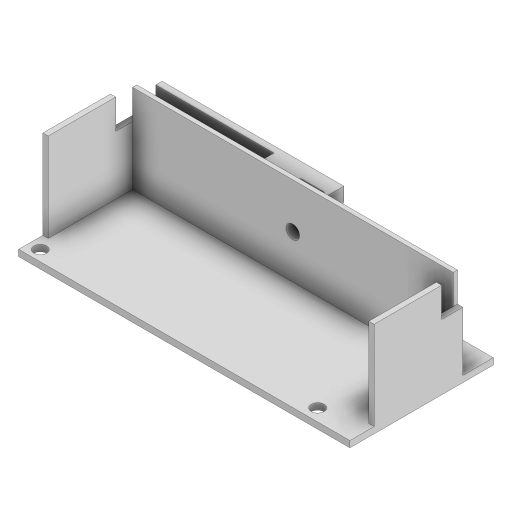
# Autodesk Inventor part: Part2
Saved by Autodesk Inventor 2023.3 (Build 273359000, 359)
## iProperties
Created: 2025-03-15
Part Number: Part2
Material: Generic
Document SubType Name: Modeling
Designer: David Zindović
Density: 1 g/cm^3
Appearance: Default
Author: David Zindović
Autodesk Inventor part; units mm, degrees
ref_plane "YZ Plane" through (0, 0, 0) normal (1, 0, 0) x (0, 1, 0)
ref_plane "XZ Plane" through (0, 0, 0) normal (0, 1, 0) x (-1, 0, 0)
sketch "Sketch1" plane through (0, 0, 0) normal (0, 0, 1) x (1, 0, 0)
  line L0 (-39.25, 11.25) -> (39.25, 11.25)
  line L1 (39.25, 11.25) -> (39.25, -11.25)
  line L2 (39.25, -11.25) -> (-39.25, -11.25)
  line L3 (-39.25, -11.25) -> (-39.25, 11.25)
  line L4 (-39.25, -11.25) -> (39.25, -11.25)
  line L5 (39.25, -11.25) -> (39.25, -9.75)
  line L6 (39.25, -9.75) -> (-39.25, -9.75)
  line L7 (-39.25, -9.75) -> (-39.25, -11.25)
  point P0 (0, 0)
  point P1 (0, 11.25)
  point P2 (39.25, 0)
  point P3 (-39.25, -9.75)
  dimension "d0" = 22.5
  dimension "d1" = 78.5
  dimension "d2" = 1.5
  constraints: 16 end point, 4 parallel, 2 horizontal, 2 midpoint, 2 perpendicular, 1 horizontal alignment, 1 point on line, 1 vertical alignment
  measures "d0" distance of L0.end L1.end
  measures "d1" distance of L1.end L2.end
  measures "d2" distance of L5.end L4.end
extrude "Extrusion1" add sketch "Sketch1" along normal blind 33 contours L6 L1 L2 L3
sketch "Sketch2" plane through (-39.25, -9.75, 0) normal (0, 1, 0) x (1, 0, 0)
  line L0 (0, -1.5) -> (28, -1.5)
  line L1 (28, -1.5) -> (28, -5.75)
  line L2 (28, -5.75) -> (0, -5.75)
  line L3 (0, -5.75) -> (0, -1.5)
  line L4 (0, 0) -> (0, -33) projected
  line L5 (78.5, 0) -> (0, 0) projected
  line L6 (0, -5.75) -> (29.5, -5.75)
  line L7 (29.5, -5.75) -> (29.5, -7.25)
  line L8 (29.5, -7.25) -> (0, -7.25)
  line L9 (0, -7.25) -> (0, -5.75)
  line L10 (0, 0) -> (78.5, 0) projected
  line L11 (29.5, -7.25) -> (28, -7.25)
  line L12 (28, -7.25) -> (28, 0)
  line L13 (28, 0) -> (29.5, 0)
  line L14 (29.5, 0) -> (29.5, -7.25)
  line L15 (0, -33) -> (78.5, -33) projected
  line L16 (1.25, -33) -> (77.25, -33)
  line L17 (77.25, -28.25) -> (77.25, -8.25)
  line L18 (77.25, -8.25) -> (1.25, -8.25)
  line L19 (1.25, -8.25) -> (1.25, -28.25)
  line L20 (0, 0) -> (0, -33) projected
  line L21 (0, -7.25) -> (78.5, -7.25)
  line L22 (78.5, 0) -> (78.5, -33) projected
  line L23 (43.075, -2.6) -> (35.425, -2.6)
  line L24 (35.425, -2.6) -> (35.425, -7.25)
  line L25 (35.425, -7.25) -> (43.075, -7.25)
  line L26 (43.075, -7.25) -> (43.075, -2.6)
  line L27 (42.075, -3.6) -> (36.425, -3.6)
  line L28 (36.425, -3.6) -> (36.425, -6.25)
  line L29 (36.425, -6.25) -> (42.075, -6.25)
  line L30 (42.075, -6.25) -> (42.075, -3.6)
  line L31 (29.5, -7.25) -> (35.425, -7.25)
  line L32 (43.075, -2.6) -> (43.075, 0)
  line L33 (77.25, -28.25) -> (1.25, -28.25)
  line L34 (77.25, -28.25) -> (78.5, -28.25)
  line L35 (1.25, -28.25) -> (0, -28.25)
  line L36 (0, -33) -> (78.5, -33)
  line L37 (78.5, -33) -> (78.5, -34)
  line L38 (78.5, -34) -> (0, -34)
  line L39 (0, -34) -> (0, -33)
  point P0 (39.25, 0)
  point P1 (39.25, -8.25)
  point P2 (39.25, 0)
  point P3 (39.25, -7.25)
  point P4 (39.25, -6.25)
  point P5 (42.075, -4.925)
  point P6 (43.075, -4.925)
  point P7 (0, -1.5)
  point P8 (0, -5.75)
  point P9 (0, -7.25)
  point P10 (0, -7.25)
  dimension "d5" = 28
  dimension "d6" = 4.25
  dimension "d7" = 1.5
  dimension "d8" = 1.5
  dimension "d9" = 1.5
  dimension "d10" = 20
  dimension "d11" = 76
  dimension "d12" = 1
  dimension "d13" = 4.65
  dimension "d14" = 7.65
  dimension "d16" = 2.65
  dimension "d17" = 5.65
  dimension "d52" = 1
  constraints: 68 end point, 14 parallel, 12 perpendicular, 8 horizontal, 7 point on line, 6 midpoint, 3 collinear, 3 vertical alignment, 1 horizontal alignment
  measures "d5" distance of L0.start L0.end
  measures "d6" distance of L0.end L1.end
  measures "d7" distance between parallel lines of L5 L0
  measures "d8" distance of L6.end L7.end
  measures "d9" distance between parallel lines of L7 L1
  measures "d10" distance of L17.start L17.end
  measures "d11" distance of L17.end L18.end
  measures "d12" distance between parallel lines of L21 L18
  measures "d13" distance of L23.end L24.end
  measures "d14" distance of L24.end L25.end
  measures "d16" distance of L27.end L28.end
  measures "d17" distance of L28.end L29.end
  measures "d52" distance of L36.end L37.end
extrude "Extrusion2" add sketch "Sketch2" along normal blind 17.5 contours L4 L5 L12 L0 | L12 L5 L14 L6 L1 | L2 L12 L8 L4 | L6 L7 L8 L12
extrude "Extrusion3" add sketch "Sketch2" along normal blind 21 contours L8 L21 L22 L34 L17 L18 L19 L35 L4
extrude "Extrusion4" add sketch "Sketch2" along normal blind 17.5 contours L14 L5 L32 L23 L24 L21 L7 | L24 L23 L26 L21
sketch "Sketch3" plane through (-38, -9.75, 8.25) normal (0, 0, 1) x (1, 0, 0)
  line L0 (75.85, 20.7) -> (0.15, 20.7)
  line L1 (0.15, 20.7) -> (0.15, 0)
  line L2 (0.15, 0) -> (75.85, 0)
  line L3 (75.85, 0) -> (75.85, 20.7)
  line L4 (76, 0) -> (0, 0) projected
  circle A0 centre (38, 10.35) radius 1.575
  line L5 (76, 0) -> (0, 0) projected
  point P0 (38, 9.75)
  point P1 (38, 20.7)
  point P2 (75.85, 10.35)
  dimension "d24" = 75.7
  dimension "d25" = 20.7
  dimension "d28" = 3.15
  constraints: 8 end point, 2 midpoint, 2 parallel, 2 vertical alignment, 1 centre point, 1 collinear, 1 horizontal, 1 horizontal alignment, 1 perpendicular
  measures "d24" distance of L0.start L0.end
  measures "d25" distance of L2.end L0.start
  measures "d28" diameter of A0
extrude "Extrusion5" [suppressed]
sketch "Sketch4" plane through (2.825, -9.75, 6.25) normal (0, 0, -1) x (-1, 0, 0)
  line L0 (5.65, 0) -> (0, 0) projected
  line L1 (5.65, 0) -> (5.65, 17.5) projected
  line L2 (0, 17.5) -> (5.65, 17.5) projected
  line L3 (0, 0) -> (0, 17.5) projected
  line L4 (2.825, 7.1746) -> (0, 8.8056)
  line L5 (0.075, 8.7623) -> (0.075, 11.9377)
  line L6 (0.075, 11.9377) -> (2.825, 13.5254)
  line L7 (2.825, 13.5254) -> (5.575, 11.9377)
  line L8 (5.575, 11.9377) -> (5.575, 8.7623)
  line L9 (5.65, 8.8056) -> (2.825, 7.1746)
  circle A0 centre (2.825, 10.35) radius 1.575
  point P0 (2.825, 9.75)
  point P1 (5.575, 10.35)
  point P2 (2.825, 0)
  dimension "d31" = 5.5
  dimension "d34" = 3.15
  dimension "d37" = 10.35
  constraints: 12 end point, 4 point on line, 2 midpoint, 2 vertical alignment, 1 centre point, 1 coincident, 13 other
  measures "d31" distance from line of point (5.575, 10.35) L5
  measures "d34" diameter of A0
  measures "d37" distance of point (2.825, 0) point (2.825, 10.35)
extrude "Extrusion6" add sketch "Sketch4" along normal up to surface (2.65 mm away) contours L0 L3 L4 L9 L1
extrude "Extrusion7" cut sketch "Sketch4" along normal mid plane 10 contours A0
fillet "Fillet1" [suppressed]
sketch "Sketch6" plane through (0, 0, 0) normal (0, 0, -1) x (-1, 0, 0)
  circle A0 centre (0, 0.6) radius 2.5
  line L0 (39.25, -11.25) -> (-39.25, -11.25) projected
  line L1 (39.25, 7.75) -> (39.25, -11.25) projected
  point P0 (0, 0)
  dimension "d43" = 5
  dimension "d44" = 11.85
  dimension "d45" = 39.25
  constraints: 1 centre point
  measures "d43" diameter of A0
  measures "d44" distance from line of A0.centre L0
  measures "d45" distance from line of L1 A0.centre
extrude "Extrusion8" cut sketch "Sketch6" against normal blind 3
chamfer "Chamfer1" distance 3 angle 45 1 edges at (2.5, 0.6, 0)
extrude "Extrusion9" add sketch "Sketch2" against normal up to surface (1.5 mm away) contours L15 L37 L38 L39
sketch "Sketch7" plane through (-11.25, -9.75, 1.5) normal (-1, 0, 0) x (0, 0, 1)
  line L0 (0.625, 9) -> (3.625, 9)
  line L1 (3.625, 9) -> (3.625, 4)
  line L2 (3.625, 4) -> (0.625, 4)
  line L3 (0.625, 4) -> (0.625, 9)
  line L4 (4.25, 0) -> (0, 0) projected
  line L5 (0, 0) -> (4.25, 0) projected
  point P0 (-1.5, 9.75)
  point P1 (2.125, 4)
  point P2 (2.125, 0)
  dimension "d55" = 4
  dimension "d56" = 3
  dimension "d57" = 5
  constraints: 8 end point, 2 midpoint, 2 parallel, 1 horizontal, 1 perpendicular, 1 vertical alignment
  measures "d55" distance between parallel lines of L2 L4
  measures "d56" distance of L1.end L2.end
  measures "d57" distance of L2.end L0.start
sketch "Sketch8" plane through (-39.25, -11.25, 0) normal (0, -1, 0) x (1, 0, 0)
  line L0 (41.75, 2) -> (36.75, 2)
  line L1 (36.75, 2) -> (36.75, 5)
  line L2 (36.75, 5) -> (41.75, 5)
  line L3 (41.75, 5) -> (41.75, 2)
  line L4 (0, 0) -> (78.5, 0) projected
  point P0 (39.25, 0)
  point P1 (39.25, 2)
  point P2 (39.25, 0)
  dimension "d58" = 5
  dimension "d59" = 3
  dimension "d60" = 2
  constraints: 8 end point, 2 midpoint, 2 parallel, 1 horizontal, 1 perpendicular, 1 vertical alignment
  measures "d58" distance of L1.end L2.end
  measures "d59" distance of L2.end L0.start
  measures "d60" distance between parallel lines of L4 L0
loft "Loft1" [suppressed]
sketch "Sketch9" plane through (39.25, 11.25, 7.25) normal (0, 0, -1) x (-1, 0, 0)
  line L0 (0, -21) -> (0, 0) projected
  line L1 (0, 0) -> (1.25, 0)
  line L2 (1.25, 0) -> (1.25, -7)
  line L3 (1.25, -7) -> (0, -7)
  line L4 (0, -7) -> (0, 0)
  line L5 (0, 0) -> (78.5, 0) projected
  point P0 (39.25, -11.25)
  point P1 (0, -7)
  dimension "d65" = 7
  constraints: 8 end point, 2 parallel, 1 coincident, 1 collinear, 1 horizontal, 1 perpendicular, 1 point on line
  measures "d65" distance of L1.end L2.end
extrude "Extrusion10" cut sketch "Sketch9" against normal blind 5
mirror "Mirror1" about plane through (0, 0, 0) normal (1, 0, 0) of "Extrusion10"
sketch "Sketch10" plane through (-39.25, -11.25, 0) normal (-1, 0, 0) x (0, 0, 1)
  line L0 (12.25, 15.5) -> (7.25, 15.5) projected
  line L1 (1.5, 19) -> (5.75, 19) projected
  line L2 (5.75, 19) -> (7.25, 19)
  line L3 (7.25, 19) -> (7.25, 15.5)
  line L4 (7.25, 15.5) -> (5.75, 15.5)
  line L5 (5.75, 15.5) -> (5.75, 19)
  point P0 (0, 11.25)
  constraints: 8 end point, 2 parallel, 1 horizontal, 1 perpendicular
extrude "Extrusion11" cut sketch "Sketch10" against normal up to surface (28 mm away)
ref_plane "Work Plane1" through (-11.25, -9.75, 3.625) normal (0, 0, -1) x (-1, 0, 0)
sketch "Sketch11" plane through (-11.25, -9.75, 3.625) normal (0, 0, -1) x (-1, 0, 0)
  line L0 (0, 0) -> (0, 14) projected
  line L1 (0, 17.5) -> (0, 14) projected
  line L2 (0, 0) -> (0, 17.5) projected
  line L3 (-15.075, 0) -> (-15.075, 6.3979) projected
  line L4 (-15.075, 6.3979) -> (-9.6656, 6.3979) construction
  line L5 (-7.5375, 0.5) -> (-16.6978, 9.6603)
  line L6 (-7.5375, 0.5) -> (5.4171, 0.5) construction
  line L7 (-15.075, 17.5) -> (0, 17.5) projected
  line L8 (-7.5375, 0.5) -> (0, 8.0375)
  line L9 (0, 0) -> (0, 14) projected
  line L10 (-7.5375, 0.5) -> (3.1221, 0.5) construction
  line L11 (-18.8191, 7.5389) -> (-7.5375, -3.7426)
  line L12 (-7.5375, -3.7426) -> (2.1213, 5.9162)
  line L13 (-49.25, 0) -> (26.75, 0) projected
  line L14 (0, 3.7949) -> (0, 8.0375)
  line L15 (-15.075, 3.7949) -> (-15.075, 8.0375)
  line L16 (-11.25, 0) -> (-11.25, -1.5)
  line L17 (-3.7949, 0) -> (-3.7949, -1.5)
  line L18 (-11.25, -1.5) -> (-3.7949, -1.5)
  line L19 (-11.25, -1.5) -> (-3.7949, -1.5)
  line L20 (-3.7949, -1.5) -> (-3.7949, -2.3604)
  line L21 (-3.7949, -2.3604) -> (-11.25, -2.3604)
  line L22 (-11.25, -2.3604) -> (-11.25, -1.5)
  line L23 (28, -1.5) -> (-50.5, -1.5) projected
  point P0 (-11.25, 9.75)
  point P1 (-7.5375, 17.5)
  point P2 (0, 3.7949)
  point P3 (0, 8.0375)
  point P4 (-11.2801, 0)
  dimension "d73" = 135
  dimension "d74" = 45
  dimension "d75" = 3
  dimension "d76" = 0.5
  constraints: 32 end point, 9 point on line, 5 horizontal, 3 midpoint, 2 equal length, 2 parallel, 2 perpendicular, 2 vertical alignment, 1 coincident, 1 vertical, 1 other
  measures "d73" angle of L6 L5
  measures "d74" angle of L10 L8
  measures "d75" distance between parallel lines of L5 L11
  measures "d76" distance from line of L13 L5.start
extrude "Extrusion12" cut sketch "Sketch11" along normal mid plane 3 contours L12 L13 L11 L3 L15 L5 L8 L0 | L17 L18 L12 | L12 L18 L11 L16 L13 | L18 L20 L21 L12 | L12 L21 L11 L18 | L18 L16 L11 | L11 L21 L22 L18
sketch "Sketch12" plane through (-38, -9.75, 8.25) normal (0, 1, 0) x (1, 0, 0)
  circle A0 centre (1.37, -23.25) radius 1.5
  line L0 (-1.25, -25.75) -> (77.25, -25.75) projected
  line L1 (-1.25, -20) -> (-1.25, -25.75) projected
  circle A1 centre (66.75, -22.875) radius 1.5
  line L2 (77.25, -20) -> (77.25, -25.75) projected
  point P0 (38, 8.25)
  dimension "d79" = 3
  dimension "d80" = 2.5
  dimension "d81" = 2.62
  dimension "d82" = 3
  dimension "d83" = 2.875
  dimension "d84" = 10.5
  constraints: 2 centre point
  measures "d79" diameter of A0
  measures "d80" distance from line of L0 A0.centre
  measures "d81" distance from line of L1 A0.centre
  measures "d82" diameter of A1
  measures "d83" distance from line of L0 A1.centre
  measures "d84" distance from line of L2 A1.centre
extrude "Extrusion13" cut sketch "Sketch12" against normal up to surface (1.5 mm away)
sketch "Sketch13" plane through (-38, -9.75, 8.25) normal (0, 1, 0) x (1, 0, 0)
  circle A0 centre (1.37, -23.25) radius 1.5 projected
  circle A1 centre (66.75, -22.875) radius 1.5 projected
  line L0 (77.25, -20) -> (76, -20) projected
  line L1 (76, -20) -> (76, 0) projected
  line L2 (76, 0) -> (0, 0) projected
  line L3 (0, 0) -> (0, -20) projected
  line L4 (0, -20) -> (-1.25, -20) projected
  line L5 (-1.25, -20) -> (-1.25, -25.75) projected
  line L6 (-1.25, -25.75) -> (77.25, -25.75) projected
  line L7 (77.25, -20) -> (77.25, -25.75) projected
  point P0 (38, 8.25)
body "Solid1"
